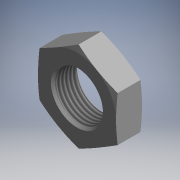
# Autodesk Inventor part: DIN-439-B - M20x1.5(F)
Saved by Autodesk Inventor 2017.3 (Build 213256000, 256)
## iProperties
Part Number: DIN-439-B - M20x1.5(F)
Material: Generic
Catalog Web Link: www.cadenas.de
Description: DIN-439 Form B-Hex nut
Vendor: FESTO
Document SubType Name: Modeling
Designer: partserver
Manufacturer: FESTO
Mass: 5.07372 g
Surface Area: 25.5009 cm^2
Volume: 5.07372 cm^3
Density: 1 g/cm^3
Appearance: PSOLRGB-192-192-192
Category: PARTsolutions
Company: FESTO
Title: DIN-439-B - M20x1.5
Author: Cadenas PARTsolutions
Comments: Hex nut
PSOL_IDENT_0: {$CADENAS_DATA\23d-libs\festo\zyl_zubeh\din_439_b\din_439_form_b.prj},190 {VTYP=3D},{NB=DIN-439-B -
PSOL_IDENT_1: M20x1.5(F)},{LINA=DIN-439-B - M20x1.5},{NN=DIN-439 Form B},{DATE=28.05.2015 11:05:12},{GEOMDATE=28.0
PSOL_IDENT_2: 5.2015 08:07:00},{VERSION=},{LINEID=200},{WBVAR=},{WBNUMERIC=}  {NB=DIN-439-B - M20x1.5(F)},{LINA=DI
PSOL_IDENT_3: N-439-B - M20x1.5},{KT=X},{IDNR=},{NENN=M20x1.5},{DG=20.000},{DK=18.376},{M=10.000},{S=30.000},{P=1.
PSOL_IDENT_4: 500}
NB: DIN-439-B - M20x1.5(F)
NN: DIN-439 Form B
NT: Hex nut
NBSYN: DIN-439-B - $NENN.(F)
LINA: DIN-439-B - M20x1.5
CATALOG: Festo
ROWDESC: M20x1.5
NENN: M20x1.5
DG: 20
DK: 18.376
M: 10
S: 30
P: 1.5
SUPPLIER: FESTO
ARTICLENO: DIN-439-B - M20x1.5(F)
BOMINFO: DIN-439-B - M20x1.5
CREATOR: CADENAS GmbH
Autodesk Inventor part; units mm, degrees
sketch "Sketch_1" plane through (0, 0, 0) normal (0, 0, 1) x (1, 0, 0)
  line L0 (0, -10) -> (0, 0)
  line L1 (0, 0) -> (14.95, 0)
  line L2 (14.95, 0) -> (33.6103, -5)
  line L3 (33.6103, -5) -> (14.95, -10)
  line L4 (14.95, -10) -> (0, -10)
  line L5 (0, -10) -> (0, 0)
  constraints: 12 end point
revolve "Revolution1" add sketch "Sketch_1" angle 360 about axis through (0, -10, 0) along (0, 1, 0)
sketch "Sketch_2" plane through (0, 0, 0) normal (0, 1, 0) x (-1, 0, 0)
  line L0 (60, -60) -> (60, 60)
  line L1 (60, 60) -> (-60, 60)
  line L2 (-60, 60) -> (-60, -60)
  line L3 (-60, -60) -> (60, -60)
  line L4 (15, 8.6603) -> (0, 17.3205)
  line L5 (0, 17.3205) -> (-15, 8.6603)
  line L6 (-15, 8.6603) -> (-15, -8.6603)
  line L7 (-15, -8.6603) -> (0, -17.3205)
  line L8 (0, -17.3205) -> (15, -8.6603)
  line L9 (15, -8.6603) -> (15, 8.6603)
  constraints: 20 end point
extrude "Extrusion1" cut sketch "Sketch_2" along normal mid plane 22
sketch "Sketch_3" plane through (0, 0, 0) normal (0, 0, 1) x (1, 0, 0)
  line L0 (0, -10) -> (0, 0)
  line L1 (0, 0) -> (10, 0)
  line L2 (10, 0) -> (9.188, -0.812)
  line L3 (9.188, -0.812) -> (9.188, -9.188)
  line L4 (9.188, -9.188) -> (10, -10)
  line L5 (10, -10) -> (0, -10)
  line L6 (0, -10) -> (0, 0)
  constraints: 14 end point
revolve "Revolution2" cut sketch "Sketch_3" angle 360 about axis through (0, -10, 0) along (0, -1, 0)
thread "Thread1" size "M20x1.5" class "6H" standard "ISO Metric profile" full length
ref_plane "2CYL_XY" through (0, -5, 0) normal (0, 1, 0) x (1, 0, 0)
ref_plane "2CYL_YZ" through (0, -5, 0) normal (1, 0, 0) x (0, 0, -1)
ref_plane "2CYL_ZX" through (0, -5, 0) normal (0, 0, -1) x (0, 1, 0)
ref_plane "din439b_punkt_XY" through (0, 0, 0) normal (0, 1, 0) x (1, 0, 0)
ref_plane "din439b_punkt_YZ" through (0, 0, 0) normal (1, 0, 0) x (0, 0, -1)
ref_plane "din439b_punkt_ZX" through (0, 0, 0) normal (0, 0, -1) x (0, 1, 0)
body "Solid1"
